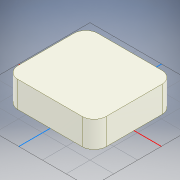
# Autodesk Inventor part: TP_LINK_MR3023
Saved by Autodesk Inventor 2022 (Build 260153000, 153)
## iProperties
Created: 2021-08-09
Part Number: TP_LINK_MR3023
Material: Типовые
Document SubType Name: Modeling
Designer: Петров Иван
Mass: 107.188 g
Surface Area: 155.706 cm^2
Volume: 107.188 cm^3
Density: 1 g/cm^3
Appearance: Гладкий — слоновая кость
Author: Петров Иван
Autodesk Inventor part; units mm, degrees
ref_plane "YZ Plane" through (0, 0, 0) normal (1, 0, 0) x (0, 1, 0)
ref_plane "XZ Plane" through (0, 0, 0) normal (0, 1, 0) x (-1, 0, 0)
ref_plane "XY Plane" through (0, 0, 0) normal (0, 0, 1) x (1, 0, 0)
sketch "Эскиз1" plane through (0, 0, 0) normal (0, 1, 0) x (-1, 0, 0)
  line L0 (-37, 33.5) -> (37, 33.5)
  line L1 (37, 33.5) -> (37, -33.5)
  line L2 (37, -33.5) -> (-37, -33.5)
  line L3 (-37, -33.5) -> (-37, 33.5)
  line L4 (-37, 33.5) -> (37, -33.5) construction
  line L5 (37, 33.5) -> (-37, -33.5) construction
  point P0 (0, 0)
  dimension "d0" = 74
  dimension "d1" = 67
  constraints: 12 end point, 2 midpoint, 2 parallel, 1 horizontal, 1 perpendicular
  measures "d0" distance of L1.end L2.end
  measures "d1" distance of L0.end L1.end
extrude "Выдавливание1" add sketch "Эскиз1" along normal blind 22
fillet "Сопряжение1" radius 10 4 edges at (-37, 11, 33.5) (37, 11, 33.5) (37, 11, -33.5) (-37, 11, -33.5)
